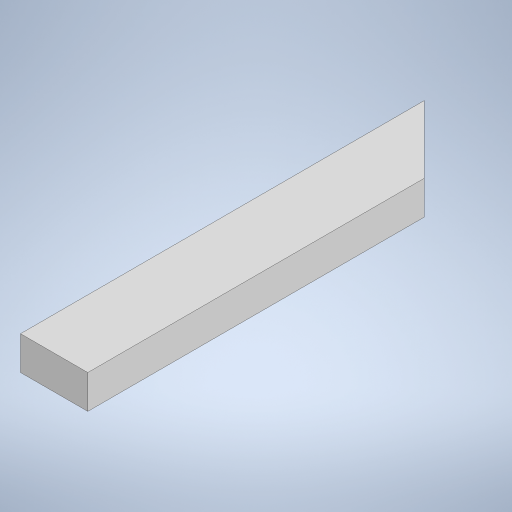
# Autodesk Inventor part: perpendicular_alum_bar
Saved by Autodesk Inventor 2024 (Build 280153000, 153)
## iProperties
Created: 2023-11-20
Part Number: perpendicular_alum_bar
Material: Generic
Document SubType Name: Modeling
Designer: s137416
Density: 1 g/cm^3
Appearance: Default
Author: s137416
Autodesk Inventor part; units mm, degrees
ref_plane "YZ Plane" through (0, 0, 0) normal (1, 0, 0) x (0, 1, 0)
ref_plane "XZ Plane" through (0, 0, 0) normal (0, 1, 0) x (-1, 0, 0)
ref_plane "XY Plane" through (0, 0, 0) normal (0, 0, 1) x (1, 0, 0)
sketch "Sketch1" plane through (0, 0, 0) normal (0, 0, 1) x (1, 0, 0)
  line L0 (-6.6363, 27.3242) -> (44.1637, 27.3242)
  line L1 (44.1637, 27.3242) -> (44.1637, 1.9242)
  line L2 (44.1637, 1.9242) -> (-6.6363, 1.9242)
  line L3 (-6.6363, 1.9242) -> (-6.6363, 27.3242)
  point P0 (0, 0)
  dimension "d0" = 50.8
  dimension "d1" = 25.4
  constraints: 8 end point, 2 parallel, 1 horizontal, 1 perpendicular
  measures "d0" distance of L1.end L2.end
  measures "d1" distance of L2.end L0.start
extrude "Extrusion1" add sketch "Sketch1" along normal blind 304.8
sketch "Sketch2" plane through (-6.6363, 1.9242, 0) normal (0, -1, 0) x (1, 0, 0)
  line L0 (0, 0) -> (50.8, 0) projected
  line L1 (0, 0) -> (50.8, 50.8)
  line L2 (50.8, 0) -> (50.8, 304.8) projected
  point P0 (6.6363, 0)
  dimension "d4" = 45
  constraints: 2 end point, 1 point on line
  measures "d4" angle of L0 L1
extrude "Extrusion2" cut sketch "Sketch2" against normal blind 304.8
body "Solid1"
